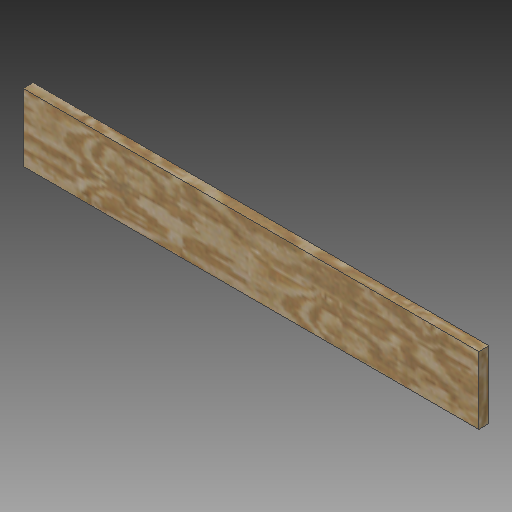
# Autodesk Inventor part: Side Board
Saved by Autodesk Inventor 2018 (Build 220112000, 112)
## iProperties
Created: 2018-01-17
Part Number: Side Board
Material: Generic
Document SubType Name: Modeling
Designer: Apple
Density: 1 g/cm^3
Appearance: Plywood - Weathered
Author: Apple
Autodesk Inventor part; units mm, degrees
ref_plane "YZ Plane" through (0, 0, 0) normal (1, 0, 0) x (0, 1, 0)
ref_plane "XZ Plane" through (0, 0, 0) normal (0, 1, 0) x (-1, 0, 0)
ref_plane "XY Plane" through (0, 0, 0) normal (0, 0, 1) x (1, 0, 0)
sketch "Sketch1" plane through (0, 0, 0) normal (0, 0, 1) x (1, 0, 0)
  line L0 (22.987, 84.3142) -> (22.987, -42.6858) projected
  line L1 (-835.787, -42.6858) -> (-835.787, 84.3142) projected
  line L2 (22.987, -42.6858) -> (-835.787, -42.6858)
  line L3 (-835.787, -42.6858) -> (-835.787, 84.3142)
  line L4 (-835.787, 84.3142) -> (22.987, 84.3142)
  line L5 (22.987, 84.3142) -> (22.987, -42.6858)
  point P0 (0, 0)
  constraints: 8 end point, 2 parallel, 1 horizontal, 1 perpendicular
extrude "Extrusion1" add sketch "Sketch1" along normal blind 19.05
body "Solid1"
